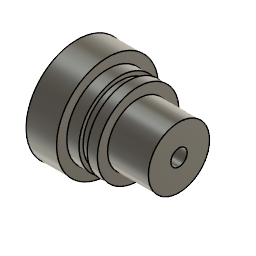
Turning_ (Autodesk Fusion 360 design; units mm, degrees)
part number: 2026-06-22-10-59-51-004
Autodesk Fusion 360 part; units mm, degrees
sketch "Sketch1" plane through (0, 0, 0) normal (0, 0, 1) x (1, 0, 0)
  line L0 (0, 0) -> (100, 0)
  line L1 (0, 0) -> (0, 50)
  line L2 (0, 50) -> (30, 50)
  line L3 (30, 50) -> (30, 40)
  line L4 (60, 40) -> (60, 30)
  line L5 (60, 30) -> (100, 30)
  line L6 (100, 30) -> (100, 0)
  line L7 (50, 40) -> (50, 36)
  line L8 (50, 36) -> (42, 36)
  line L9 (42, 36) -> (42, 40)
  line L10 (30, 40) -> (42, 40)
  line L11 (50, 40) -> (60, 40)
  dimension "d1" = 100
  dimension "d2" = 50
  dimension "d3" = 4
  dimension "d4" = 8
  constraint coincident L0.start L1.start
  constraint horizontal L0
  constraint perpendicular L0 L1
  constraint perpendicular L1 L2
  constraint perpendicular L2 L3
  constraint perpendicular L3 L10
  constraint perpendicular L4 L11
  constraint perpendicular L3 L5
  constraint perpendicular L0 L6
  constraint vertical L7
  constraint horizontal L8
  constraint vertical L9
  constraint collinear L10 L11
  measures "d1" distance of L0.start L0.end
  measures "d2" distance of L0.start L1.end
  measures "d3" distance of L9.end L8.end
  measures "d4" distance of L7.end L8.end
revolve "Revolve1" add sketch "Sketch1" angle 360 about axis through (0, 0, 0) along (1, 0, 0)
sketch "Sketch2" plane through (100, 0, 0) normal (1, 0, 0) x (0, 1, 0)
  circle A0 centre (0, 0) radius 30
hole "Hole1" at (100, 0, 0) direction (-1, 0, 0) diameter 16 end through all
